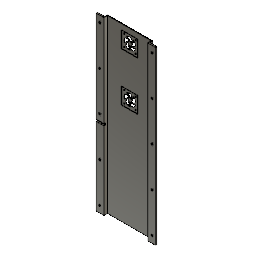
1-CBA_bottom_Cover_V3_Full v1 (Autodesk Fusion 360 design; units mm, degrees)
Autodesk Fusion 360 part; units mm, degrees
sketch "Main Profile" plane through (0, 0, 0) normal (0, 0, 1) x (1, 0, 0)
  line L0 (-62.5, 0) -> (62.5, 0)
  line L1 (62.5, 0) -> (62.5, -8)
  line L2 (62.5, -8) -> (82.5, -8)
  line L3 (82.5, -8) -> (82.5, -12)
  line L4 (82.5, -12) -> (60.5, -12)
  line L5 (60.5, -12) -> (60.5, -2)
  line L6 (60.5, -2) -> (-60.5, -2)
  line L7 (0, -2) -> (0, 0) construction
  line L8 (-62.5, 0) -> (-62.5, -8)
  line L9 (-62.5, -8) -> (-82.5, -8)
  line L10 (-82.5, -8) -> (-82.5, -12)
  line L11 (-82.5, -12) -> (-60.5, -12)
  line L12 (-60.5, -12) -> (-60.5, -2)
  dimension "d1" = 125
  dimension "d2" = 8
  dimension "d3" = 20
  dimension "d4" = 4
  dimension "d5" = 2
  dimension "d6" = 2
  constraint horizontal L0
  constraint midpoint L7.end L0
  constraint perpendicular L0 L1
  constraint perpendicular L1 L2
  constraint perpendicular L0 L3
  constraint perpendicular L3 L4
  constraint perpendicular L0 L5
  constraint perpendicular L5 L6
  constraint midpoint L6 L7.start
  constraint coincident L7.end origin
  constraint vertical L7
  constraint symmetric L0.end L7 L0.start
  constraint symmetric L1.end L7 L8.end
  constraint symmetric L2.end L7 L9.end
  constraint symmetric L3.end L7 L10.end
  constraint symmetric L4.end L7 L11.end
  constraint symmetric L5.end L7 L6.end
  measures "d1" distance of L0.start L0.end
  measures "d2" distance of L0.end L1.end
  measures "d3" distance of L1.end L2.end
  measures "d4" distance of L2.end L3.end
  measures "d5" distance of L1 L5
  measures "d6" distance of L0 L6
extrude "Extrude1" add sketch "Main Profile" along normal blind 475
sketch "Holes and Fans" plane through (0, -12, 0) normal (0, -1, 0) x (1, 0, 0)
  line L0 (-82.5, 0) -> (-60.5, 0)
  line L1 (-60.5, 0) -> (-60.5, 475)
  line L2 (-60.5, 475) -> (-82.5, 475)
  line L3 (-82.5, 475) -> (-82.5, 0)
  circle A0 centre (-72.5, 19) radius 2.75
  circle A1 centre (72.5, 19) radius 2.75
  circle A2 centre (-72.5, 128.5) radius 2.75
  circle A3 centre (72.5, 128.5) radius 2.75
  circle A4 centre (-72.5, 238) radius 2.75
  circle A5 centre (72.5, 238) radius 2.75
  circle A6 centre (-72.5, 347.5) radius 2.75
  circle A7 centre (72.5, 347.5) radius 2.75
  circle A8 centre (-72.5, 457) radius 2.75
  circle A9 centre (72.5, 457) radius 2.75
  line L4 (-60.5, 220.5) -> (-82.5, 220.5)
  line L5 (-60.5, 0) -> (-60.5, 475)
  line L6 (-82.5, 215.5) -> (-60.5, 215.5)
  line L7 (-62.5, 0) -> (62.5, 0)
  circle A10 centre (-72.5, 19) radius 5
  circle A11 centre (72.5, 19) radius 5
  circle A12 centre (-72.5, 128.5) radius 5
  circle A13 centre (72.5, 128.5) radius 5
  circle A14 centre (-72.5, 238) radius 5
  circle A15 centre (72.5, 238) radius 5
  circle A16 centre (-72.5, 347.5) radius 5
  circle A17 centre (72.5, 347.5) radius 5
  circle A18 centre (-72.5, 457) radius 5
  circle A19 centre (72.5, 457) radius 5
  line L8 (-22.5, 279.5) -> (22.5, 279.5)
  line L9 (22.5, 279.5) -> (22.5, 324.5)
  line L10 (22.5, 324.5) -> (-22.5, 324.5)
  line L11 (-22.5, 324.5) -> (-22.5, 279.5)
  line L12 (-22.5, 279.5) -> (22.5, 324.5) construction
  line L13 (22.5, 279.5) -> (-22.5, 324.5) construction
  circle A20 centre (-16, 318) radius 1.75
  arc A21 (-14.6568, 308.0301) -> (-14.8488, 296.4291) centre (0.0725, 301.9843) ccw
  arc A22 (-0.5312, 306.337) -> (-14.6568, 308.0301) centre (-8.5191, 299.4657) ccw
  arc A23 (-0.5312, 306.337) -> (-14.8488, 296.4291) centre (0.559, 289.4626) ccw
  arc A24 (-4.2888, 302.835) -> (-10.2642, 289.9239) centre (-0.2223, 293.1147) ccw
  arc A25 (-10.2642, 289.9239) -> (0.7098, 286.1565) centre (0.0373, 302.0641) ccw
  arc A26 (-4.2888, 302.835) -> (0.7098, 286.1565) centre (12.0965, 298.6574) ccw
  arc A27 (-2.1195, 298.1791) -> (8.3132, 288.5065) centre (8.3817, 299.0429) ccw
  arc A28 (8.3132, 288.5065) -> (15.2874, 297.7791) centre (-0.0495, 302.0553) ccw
  arc A29 (-2.1195, 298.1791) -> (15.2874, 297.7791) centre (6.917, 312.4715) ccw
  arc A30 (2.9789, 298.8035) -> (15.4021, 305.7366) centre (5.4025, 309.0577) ccw
  arc A31 (15.4021, 305.7366) -> (8.7384, 315.2349) centre (-0.0679, 301.9701) ccw
  arc A32 (2.9789, 298.8035) -> (8.7384, 315.2349) centre (-7.8216, 311.8143) ccw
  arc A33 (3.9606, 303.8454) -> (1.2058, 317.8029) centre (-5.0428, 309.319) ccw
  arc A34 (1.2058, 317.8029) -> (-9.8868, 314.4005) centre (0.0075, 301.9262) ccw
  arc A35 (3.9606, 303.8454) -> (-9.8868, 314.4005) centre (-11.751, 297.5941) ccw
  circle A36 centre (-15.9941, 286.1048) radius 1.75
  circle A37 centre (15.9011, 286.1107) radius 1.75
  circle A38 centre (15.8952, 318.0059) radius 1.75
  line L14 (-22.5, 459.5) -> (-22.5, 414.5)
  line L15 (-22.5, 414.5) -> (22.5, 414.5)
  line L16 (22.5, 414.5) -> (22.5, 459.5)
  line L17 (22.5, 459.5) -> (-22.5, 459.5)
  circle A39 centre (15.8952, 453.0059) radius 1.75
  circle A40 centre (15.9011, 421.1107) radius 1.75
  circle A41 centre (-15.9941, 421.1048) radius 1.75
  circle A42 centre (-16, 453) radius 1.75
  arc A43 (-0.5312, 441.337) -> (-14.6568, 443.0301) centre (-8.5191, 434.4657) ccw
  arc A44 (-14.6568, 443.0301) -> (-14.8488, 431.4291) centre (0.0725, 436.9843) ccw
  arc A45 (-0.5312, 441.337) -> (-14.8488, 431.4291) centre (0.559, 424.4626) ccw
  arc A46 (-4.2888, 437.835) -> (-10.2642, 424.9239) centre (-0.2223, 428.1147) ccw
  arc A47 (-10.2642, 424.9239) -> (0.7098, 421.1565) centre (0.0373, 437.0641) ccw
  arc A48 (-4.2888, 437.835) -> (0.7098, 421.1565) centre (12.0965, 433.6574) ccw
  arc A49 (-2.1195, 433.1791) -> (8.3132, 423.5065) centre (8.3817, 434.0429) ccw
  arc A50 (-2.1195, 433.1791) -> (15.2874, 432.7791) centre (6.917, 447.4715) ccw
  arc A51 (8.3132, 423.5065) -> (15.2874, 432.7791) centre (-0.0495, 437.0553) ccw
  arc A52 (2.9789, 433.8035) -> (15.4021, 440.7366) centre (5.4025, 444.0577) ccw
  arc A53 (15.4021, 440.7366) -> (8.7384, 450.2349) centre (-0.0679, 436.9701) ccw
  arc A54 (2.9789, 433.8035) -> (8.7384, 450.2349) centre (-7.8216, 446.8143) ccw
  arc A55 (3.9606, 438.8454) -> (1.2058, 452.8029) centre (-5.0428, 444.319) ccw
  arc A56 (3.9606, 438.8454) -> (-9.8868, 449.4005) centre (-11.751, 432.5941) ccw
  arc A57 (1.2058, 452.8029) -> (-9.8868, 449.4005) centre (0.0075, 436.9262) ccw
  point P0 (0, 302)
  dimension "d9" = 5.5
  dimension "d10" = 19
  dimension "d11" = 10
  dimension "d14" = 145
  dimension "d15" = 109.5
  dimension "d16" = 5
  dimension "d17" = 215.5
  dimension "d22" = 10
  dimension "d26" = 45
  dimension "d27" = 45
  dimension "d28" = 279.5
  dimension "d29" = 3.5
  dimension "d30" = 16
  dimension "d32" = 360
  dimension "d34" = 360
  dimension "d37" = 0
  dimension "d38" = 135
  constraint coincident L1 L4.start
  constraint perpendicular L1 L4
  constraint coincident L3 L4.end
  constraint coincident L3 L6.start
  constraint coincident L5 L6.end
  constraint perpendicular L3 L6
  constraint concentric A0 A10
  constraint perpendicular L8 L9
  constraint parallel L8 L10
  constraint parallel L9 L11
  constraint horizontal L8
  constraint coincident L12 P0
  constraint coincident L13 P0
  constraint vertical origin P0
  constraint coincident L13 A20.centre
  measures "d9" diameter of A0
  measures "d10" distance of L0 A0.centre
  measures "d11" distance of L3 A0.centre
  measures "d16" distance of L4 L6
  measures "d17" distance of L6 L7
  measures "d22" diameter of A10
  measures "d26" distance of L9.end L10.end
  measures "d27" distance of L8.end L9.end
  measures "d28" distance of origin L8
  measures "d29" diameter of A20
  measures "d30" horizontal distance of P0 A20.centre
extrude "Extrude5" cut sketch "Holes and Fans" against normal blind 50 contours A20 | A21 A22 A23 | A24 A25 A26 | A27 A28 A29 | A30 A31 A32 | A33 A34 A35 | A36 | A37 | A38 | A39 | A40 | A41 | A42 | A43 A44 A45 | A46 A47 A48 | A49 A50 A51 | A52 A53 A54 | A55 A56 A57
extrude "Extrude2" cut sketch "Holes and Fans" against normal blind 20 contours A0 | A1 | A2 | A3 | A4 | A5 | A6 | A7 | A8 | A9
extrude "Extrude4" cut sketch "Holes and Fans" against normal blind 2 from surface at -2 contours A10 | A11 | A12 | A13 | A14 | A15 | A16 | A17 | A18 | A19
extrude "Extrude3" cut sketch "Holes and Fans" against normal blind 4 contours L1 L3 L4 L5 L6
extrude "Extrude6" cut sketch "Holes and Fans" against normal blind 11 contours L8 L9 L10 L11 | L14 L15 L16 L17
fillet "Fillet1" radius 0.8 10 edges at (-2.1195, -0.5, 298.1791) (-4.2888, -0.5, 302.835) (-0.5312, -0.5, 306.337) (3.9606, -0.5, 303.8454) (2.9789, -0.5, 298.8035) (-2.1195, -0.5, 433.1791) (-4.2888, -0.5, 437.835) (-0.5312, -0.5, 441.337) (3.9606, -0.5, 438.8454) (2.9789, -0.5, 433.8035)
named bodies: "1-CBA bottom Cover V3 Full"
